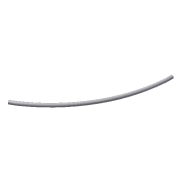
# Autodesk Inventor part: 2f2arc
Saved by Autodesk Inventor 2016 (Build 200138000, 138)
## iProperties
Company: HERA Project
Created: 2013-07-11
Part Number: 2f2arc
Material: Generic
Document SubType Name: Modeling
Designer: Dave
Density: 1 g/cm^3
Description: feed backplane pvc arc
Mass: 134.142 g
Surface Area: 939.016 cm^2
Volume: 134.142 cm^3
Appearance: Default
Author: David DeBoer
Autodesk Inventor part; units mm, degrees
ref_plane "YZ Plane" through (0, 0, 0) normal (1, 0, 0) x (0, 1, 0)
ref_plane "XZ Plane" through (0, 0, 0) normal (0, 1, 0) x (-1, 0, 0)
ref_plane "XY Plane" through (0, 0, 0) normal (0, 0, 1) x (1, 0, 0)
sketch "Sketch1" plane through (0, 0, 0) normal (0, 0, 1) x (1, 0, 0)
  circle A0 centre (596.9, -0.0117) radius 11
  line L0 (-252.1, 80.9625) -> (-252.1, -95.25)
  circle A1 centre (596.9, -0.0117) radius 9.38
  dimension "d6" = 22
  dimension "d7" = 849
  dimension "d9" = 1.62
  constraints: 2 centre point, 2 end point, 1 coincident, 1 vertical
  measures "d6" diameter of A0
  measures "d7" distance from line of L0 A0.centre
  measures "d9" radial gap between concentric circles of A1 A0
revolve "Revolution1" add sketch "Sketch1" angle 60 about axis through (-252.1, 80.9625, 0) along (0, -1, 0)
sketch "Sketch4" plane through (0, 0, 0) normal (0, 1, 0) x (-1, 0, 0)
  line L0 (-607.9, 0) -> (-585.9, 0) projected
  line L1 (-607.9, 0) -> (252.1, 0) construction
  line L2 (252.1, 0) -> (-595.0871, 55.4533) construction
  line L3 (-177.9, 744.7818) -> (-166.9, 725.7293) projected
  line L4 (252.1, 0) -> (-177.9, 744.7818) construction
  line L5 (252.1, 0) -> (-225.628, 715.1056) construction
  arc A0 (-177.9, 744.7818) -> (-607.9, 0) centre (252.1, 0) ccw projected
  arc A1 (-595.0871, 55.4533) -> (-596.9, 0) centre (252.1, 0) ccw
  arc A2 (-172.4, 735.2556) -> (-219.5175, 705.9589) centre (252.1, 0) ccw
  point P0 (0, 0)
  dimension "d10" = 860
  dimension "d12" = 3.745
  dimension "d13" = 3.745
  constraints: 8 end point, 5 point on circle, 3 point on line, 2 centre point, 1 coincident, 1 collinear
  measures "d10" distance of L0.start L1.end
  measures "d12" angle of L1 L2
  measures "d13" angle of L4 L5
sketch "Sketch5" plane through (596.9, -0.0117, 0) normal (0, 0, -1) x (-1, 0, 0)
  circle A0 centre (0, 0) radius 9.38
  circle A1 centre (0, 0) radius 11
  point P0 (596.9, 0.0117)
  constraints: 2 centre point, 1 coincident
sweep "Sweep1" cut profiles "Sketch5" path "Sketch4" path curves A1
sketch "Sketch6" plane through (172.4, -0.0117, 735.2556) normal (-0.8660254, 0, 0.5) x (0.5, 0, 0.8660254)
  circle A0 centre (0, 0) radius 9.38
  circle A1 centre (0, 0) radius 11
  point P0 (-722.95, 0.0117)
  constraints: 2 centre point, 1 coincident
sweep "Sweep2" cut profiles "Sketch6" path "Sketch4" path curves A2
sketch "Sketch11" plane through (0, 0, 0) normal (0, 1, 0) x (-1, 0, 0)
  line L0 (-225.628, 715.1056) -> (-213.407, 696.8122) projected
  line L1 (-219.5175, 705.9589) -> (-185.3078, 725.7059)
  line L2 (-584.1106, 54.7348) -> (-606.0636, 56.1718) projected
  line L3 (-595.0871, 55.4533) -> (-595.0836, 15.9533)
  point P0 (0, 0)
  dimension "d26" = 39.5
  dimension "d32" = 93.75
  dimension "d33" = 39.5
  dimension "d34" = 93.75
  constraints: 4 end point, 2 midpoint
  measures "d26" distance of L1.start L1.end
  measures "d32" angle of L0 L1
  measures "d33" distance of L3.start L3.end
  measures "d34" angle of L2 L3
sketch "Sketch12" plane through (219.5175, -0.0117, 705.9589) normal (-0.8315181, 0, 0.5554977) x (0.5554977, 0, 0.8315181)
  circle A0 centre (0, 0) radius 9.2599
  circle A1 centre (0, 0) radius 11
  point P0 (-708.959, 0.0117)
  constraints: 2 centre point, 1 coincident
sweep "Sweep4" add profiles "Sketch12" path "Sketch11" path curves L1
sketch "Sketch13" plane through (595.0871, -0.0117, 55.4533) normal (0.065316, 0, -0.9978646) x (-0.9978646, 0, -0.065316)
  circle A0 centre (0, 0) radius 9.38
  circle A1 centre (0, 0) radius 11
  point P0 (597.4383, 0.0117)
  constraints: 2 centre point, 1 coincident
sweep "Sweep5" add profiles "Sketch13" path "Sketch11" path curves L3
body "Solid1"
